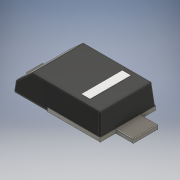
# Autodesk Inventor part: Semiconductor_POWERMITE
Saved by Autodesk Inventor 2018 (Build 220112000, 112)
## iProperties
Created: 2018-09-29
Part Number: Semiconductor_POWERMITE
Material: ABS Plastic
Document SubType Name: Modeling
Designer: Bradley
Density: 1.06 g/cm^3
Appearance: Smooth - Black
Author: Bradley
Autodesk Inventor part; units mm, degrees
ref_plane "YZ Plane" through (0, 0, 0) normal (1, 0, 0) x (0, 1, 0)
ref_plane "XZ Plane" through (0, 0, 0) normal (0, 1, 0) x (-1, 0, 0)
ref_plane "XY Plane" through (0, 0, 0) normal (0, 0, 1) x (1, 0, 0)
sketch "Sketch2" plane through (0, 0, 0) normal (0, 0, 1) x (1, 0, 0)
  line L0 (-0.9, 0.95) -> (0.9, 0.95)
  line L1 (0.9, 0.95) -> (0.9, -0.95)
  line L2 (0.9, -0.95) -> (-0.9, -0.95)
  line L3 (-0.9, -0.95) -> (-0.9, 0.95)
  line L4 (0.9, 0.425) -> (1.5, 0.425)
  line L5 (1.5, 0.425) -> (1.5, -0.425)
  line L6 (1.5, -0.425) -> (0.9, -0.425)
  line L7 (0.9, -0.425) -> (0.9, 0.425)
  line L8 (-2.3, 0.275) -> (-1.75, 0.275)
  line L9 (-1.75, 0.275) -> (-1.75, -0.275)
  line L10 (-1.75, -0.275) -> (-2.3, -0.275)
  line L11 (-2.3, -0.275) -> (-2.3, 0.275)
  line L12 (-0.9, 0) -> (0.9, 0) construction
  point P0 (0, 0)
  point P1 (-1.75, 0)
  point P2 (0, 0)
  dimension "d4" = 0.85
  dimension "d5" = 2.4
  dimension "d6" = 0.6
  dimension "d7" = 1.9
  dimension "d8" = 3.8
  dimension "d9" = 0.55
  dimension "d10" = 0.55
  constraints: 26 end point, 6 parallel, 5 midpoint, 4 horizontal, 3 horizontal alignment, 3 perpendicular, 1 coincident, 1 point on line
  measures "d4" distance of L4.end L5.end
  measures "d5" distance between parallel lines of L5 L3
  measures "d6" distance of L4.start L4.end
  measures "d7" distance of L2.end L0.start
  measures "d8" distance between parallel lines of L11 L5
  measures "d9" distance of L8.start L8.end
  measures "d10" distance of L10.end L8.start
extrude "Extrusion2" add sketch "Sketch2" along normal mid plane 0.15
sketch "Sketch3" plane through (0, 0, 0) normal (0, 0, 1) x (1, 0, 0)
  line L0 (-2.05, 0.95) -> (0.9, 0.95)
  line L1 (0.9, 0.95) -> (0.9, -0.95)
  line L2 (0.9, -0.95) -> (-2.05, -0.95)
  line L3 (-2.05, -0.95) -> (-2.05, 0.95)
  line L4 (0.9, -0.425) -> (1.5, -0.425) projected
  line L5 (1.5, -0.425) -> (1.5, 0.425) projected
  line L6 (1.5, 0.425) -> (0.9, 0.425) projected
  line L7 (0.9, 0.425) -> (0.9, 0.95) projected
  line L8 (0.9, 0.95) -> (-0.9, 0.95) projected
  line L9 (-0.9, 0.95) -> (-0.9, -0.95) projected
  line L10 (-0.9, -0.95) -> (0.9, -0.95) projected
  line L11 (0.9, -0.95) -> (0.9, -0.425) projected
  line L12 (-1.75, 0.275) -> (-2.3, 0.275) projected
  line L13 (-2.3, 0.275) -> (-2.3, -0.275) projected
  line L14 (-2.3, -0.275) -> (-1.75, -0.275) projected
  line L15 (-1.75, -0.275) -> (-1.75, 0.275) projected
  line L16 (0.9, 0.95) -> (-0.9, 0.95) projected
  line L17 (-0.9, -0.95) -> (0.9, -0.95) projected
  line L18 (0.9, 0.425) -> (0.9, 0.95) projected
  point P0 (0, 0)
  dimension "d13" = 2.95
  constraints: 8 end point, 3 collinear, 2 parallel, 1 horizontal, 1 perpendicular
  measures "d13" distance of L0.start L0.end
sketch "Sketch3 outline for Extrusion3" plane through (0, 0, 0) normal (0, 0, 1) x (1, 0, 0)
  line L0 (-2.05, 0.95) -> (0.9, 0.95)
  line L1 (0.9, 0.95) -> (0.9, -0.95)
  line L2 (0.9, -0.95) -> (-2.05, -0.95)
  line L3 (-2.05, -0.95) -> (-2.05, 0.95)
extrude "Extrusion3" add sketch "Sketch3 outline for Extrusion3" along normal blind 0.78 draft -5 and the other way blind 0.07 draft -5
chamfer "Chamfer1" distance 0.5 angle 45 1 edges at (-1.9818, 0, 0.78)
sketch "Sketch4" plane through (0, 0, 0.78) normal (0, 0, 1) x (1, 0, 0)
  line L0 (0.3, 0.7) -> (0, 0.7)
  line L1 (0, 0.7) -> (0, -0.7)
  line L2 (0, -0.7) -> (0.3, -0.7)
  line L3 (0.3, -0.7) -> (0.3, 0.7)
  point P0 (0, 0)
  point P1 (0, 0)
  dimension "d21" = 0.3
  dimension "d22" = 1.4
  constraints: 8 end point, 2 parallel, 1 coincident, 1 horizontal, 1 midpoint, 1 perpendicular
  measures "d21" distance of L0.start L0.end
  measures "d22" distance of L0.end L1.end
extrude "Extrusion4" add sketch "Sketch4" along normal blind 0.01
fillet "Fillet1" radius 0.05 17 edges at (-1.7535, 0.9035, 0.531) (-0.325, 0.8818, 0.78) (-1.4818, 0, 0.78) (-0.325, -0.8818, 0.78) (0.8318, 0, 0.78) (0.8626, -0.9126, 0.4275) (0.8626, 0.9126, 0.4275) (-1.7535, -0.9035, 0.531) (-2.0253, 0, 0.2819) (-2.0377, -0.9377, 0.141) (-2.0469, -0.9469, -0.035) (-2.0439, -0.6094, -0.07) (-1.4719, -0.9439, -0.07) (-2.0377, 0.9377, 0.141) (-2.0469, 0.9469, -0.035) (-2.0439, 0.6094, -0.07) (-1.4719, 0.9439, -0.07)
fillet "Fillet2" radius 0.02 26 edges at (0, 0.95, -0.075) (-2.025, 0.275, -0.075) (-2.1717, 0.275, 0.075) (-2.3, 0, 0.075) (-2.1717, -0.275, 0.075) (-2.3, -0.275, 0) (-2.3, 0, -0.075) (-2.3, 0.275, 0) (-1.75, 0, -0.075) (0.9, 0.425, 0) (1.2, 0.425, 0.075) (1.2, 0.425, -0.075) (0.9, 0.6875, -0.075) (1.5, 0.425, 0) (1.5, 0, 0.075) (1.5, 0, -0.075) (1.5, -0.425, 0) (1.2, -0.425, 0.075) (1.2, -0.425, -0.075) (0.9, -0.425, 0) (0.9, -0.6875, -0.075) (0.9, -0.95, 0) (0, -0.95, -0.075) (-0.9, 0, -0.075) (0.9, 0.95, 0) (-2.025, -0.275, -0.075)
body "Solid2"
